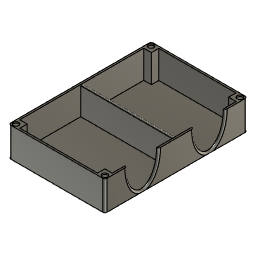
Wingspan - Birdcards (Autodesk Fusion 360 design; units mm, degrees)
Autodesk Fusion 360 part; units mm, degrees
sketch "Skizze1" plane through (0, 0, 0) normal (0, 0, 1) x (1, 0, 0)
  line L0 (0, 0) -> (91.5, 0)
  line L1 (91.5, 0) -> (91.5, 135.5)
  line L2 (91.5, 135.5) -> (0, 135.5)
  line L3 (0, 135.5) -> (0, 0)
  line L4 (1.75, 126.75) -> (89.75, 126.75)
  line L5 (89.75, 126.75) -> (89.75, 68.75)
  line L6 (89.75, 68.75) -> (1.75, 68.75)
  line L7 (1.75, 68.75) -> (1.75, 126.75)
  line L8 (0, 135.5) -> (7, 135.5)
  line L9 (7, 135.5) -> (7, 128.5)
  line L10 (7, 128.5) -> (0, 128.5)
  line L11 (0, 128.5) -> (0, 135.5)
  circle A0 centre (3.5, 132) radius 2.65
  line L12 (1.75, 66.75) -> (89.75, 66.75)
  line L13 (89.75, 66.75) -> (89.75, 8.75)
  line L14 (89.75, 8.75) -> (1.75, 8.75)
  line L15 (1.75, 8.75) -> (1.75, 66.75)
  line L16 (0, 0) -> (7, 0)
  line L17 (7, 0) -> (7, 7)
  line L18 (7, 7) -> (0, 7)
  line L19 (0, 7) -> (0, 0)
  circle A1 centre (3.5, 3.5) radius 2.65
  line L20 (91.5, 0) -> (84.5, 0)
  line L21 (84.5, 0) -> (84.5, 7)
  line L22 (84.5, 7) -> (91.5, 7)
  line L23 (91.5, 7) -> (91.5, 0)
  circle A2 centre (88, 3.5) radius 2.65
  line L24 (91.5, 135.5) -> (84.5, 135.5)
  line L25 (84.5, 135.5) -> (84.5, 128.5)
  line L26 (84.5, 128.5) -> (91.5, 128.5)
  line L27 (91.5, 128.5) -> (91.5, 135.5)
  circle A3 centre (88, 132) radius 2.65
  line L28 (9, 126.75) -> (82.5, 126.75)
  line L29 (82.5, 126.75) -> (82.5, 133.75)
  line L30 (82.5, 133.75) -> (9, 133.75)
  line L31 (9, 133.75) -> (9, 126.75)
  line L32 (8.75, 8.75) -> (82.75, 8.75)
  line L33 (82.75, 8.75) -> (82.75, 1.75)
  line L34 (82.75, 1.75) -> (8.75, 1.75)
  line L35 (8.75, 1.75) -> (8.75, 8.75)
  dimension "d3" = 88
  dimension "d4" = 58
  dimension "d5" = 7
  dimension "d6" = 7
  dimension "d7" = 5.3
  dimension "d9" = 3.5
  dimension "d10" = 3.5
  dimension "d11" = 1.75
  dimension "d12" = 1.75
  dimension "d13" = 88
  dimension "d14" = 58
  dimension "d15" = 2
  dimension "d16" = 1.75
  dimension "d17" = 8.75
  dimension "d18" = 8.75
  dimension "d19" = 135.5
  dimension "d20" = 7
  dimension "d21" = 7
  dimension "d22" = 5.3
  dimension "d24" = 3.5
  dimension "d25" = 3.5
  dimension "d26" = 1.75
  dimension "d27" = 7
  dimension "d28" = 7
  dimension "d29" = 5.3
  dimension "d30" = 3.5
  dimension "d32" = 3.5
  dimension "d33" = 7
  dimension "d34" = 7
  dimension "d35" = 5.3
  dimension "d36" = 3.5
  dimension "d37" = 3.5
  dimension "d38" = 2
  dimension "d39" = 2
  dimension "d40" = 1.75
  dimension "d41" = 1.75
  dimension "d42" = 1.75
  dimension "d43" = 1.75
  constraint horizontal L0
  constraint vertical L1
  constraint horizontal L2
  constraint vertical L3
  constraint coincident L0.start L3.end
  constraint horizontal L4
  constraint vertical L5
  constraint horizontal L6
  constraint vertical L7
  constraint horizontal L8
  constraint vertical L9
  constraint horizontal L10
  constraint vertical L11
  constraint horizontal L12
  constraint vertical L13
  constraint horizontal L14
  constraint vertical L15
  constraint horizontal L16
  constraint vertical L17
  constraint horizontal L18
  constraint vertical L19
  constraint horizontal L20
  constraint vertical L21
  constraint horizontal L22
  constraint vertical L23
  constraint horizontal L24
  constraint vertical L25
  constraint horizontal L26
  constraint vertical L27
  constraint horizontal L28
  constraint vertical L29
  constraint horizontal L30
  constraint vertical L31
  constraint coincident L4 L28.start
  constraint horizontal L32
  constraint vertical L33
  constraint horizontal L34
  constraint vertical L35
  constraint coincident L14 L32.start
  measures "d3" distance of L4.start L4.end
  measures "d4" distance of L4.start L6.end
  measures "d5" distance of L2.end L8.end
  measures "d6" distance of L2.end L10.end
  measures "d7" diameter of A0
  measures "d9" distance of L10 A0.centre
  measures "d10" distance of L11 A0.centre
  measures "d11" distance of L3 L7
  measures "d12" distance of L4 L10
  measures "d13" distance of L12.start L12.end
  measures "d14" distance of L12.start L14.end
  measures "d16" distance of L3 L15
  measures "d17" distance of L2 L4
  measures "d18" distance of L0 L14
  measures "d19" distance of L0 L2
  measures "d20" distance of L0.start L16.end
  measures "d21" distance of L0.start L18.end
  measures "d22" diameter of A1
  measures "d24" distance of L16 A1.centre
  measures "d25" distance of L3 A1.centre
  measures "d26" distance of L1 L13
  measures "d27" distance of L0.end L20.end
  measures "d28" distance of L0.end L22.end
  measures "d29" diameter of A2
  measures "d30" distance of L1 A2.centre
  measures "d32" distance of L0 A2.centre
  measures "d33" distance of L1.end L24.end
  measures "d34" distance of L1.end L26.end
  measures "d35" diameter of A3
  measures "d36" distance of L24 A3.centre
  measures "d37" distance of L27 A3.centre
  measures "d38" distance of L9 L31
  measures "d39" distance of L25 L29
  measures "d40" distance of L2 L30
  measures "d41" distance of L0 L34
  measures "d42" distance of L17 L35
  measures "d43" distance of L21 L33
sketch "Skizze2" plane through (0, 0, 0) normal (0, 0, 1) x (1, 0, 0)
  line L0 (0, 0) -> (91.5, 0)
  line L1 (91.5, 0) -> (91.5, 135.5)
  line L2 (91.5, 135.5) -> (0, 135.5)
  line L3 (0, 135.5) -> (0, 0)
  dimension "d44" = 91.5
  dimension "d45" = 135.5
  constraint horizontal L0
  constraint vertical L1
  constraint horizontal L2
  constraint vertical L3
  constraint coincident L0.start L3.end
  measures "d44" distance of L0.start L0.end
  measures "d45" distance of L0.start L2.end
extrude "Extrusion7" add sketch "Skizze2" against normal blind 28
extrude "Extrusion8" cut sketch "Skizze1" against normal blind 26.5 contours L4 L5 L6 L7 L28 | L4 L28 L29 L30 L31 | L12 L13 L14 L15 L32 | L14 L32 L33 L34 L35
extrude "Extrusion9" cut sketch "Skizze1" against normal blind 1.1 contours A0 | A1 | A2 | A3
extrude "Extrusion11" cut 3 faces at (87.1265, 132.8635, -1.1) (3.4053, 132.6906, -1.1) (88.066, 2.6191, -1.1) along direction (0, 0, -1) blind 0.1
sketch "Skizze5" plane through (91.5, 0, 0) normal (1, 0, 0) x (0, 1, 0)
  line L0 (135.5, 0) -> (0, 0)
  line L1 (0, 0) -> (0, -28)
  line L2 (0, -28) -> (135.5, -28)
  line L3 (135.5, -28) -> (135.5, 0)
  ellipse E0 centre (36, 0) end of major axis (51, 0) minor radius 26.5
  line L4 (21, 0) -> (51, 0)
  line L5 (36, -26.5) -> (36, 26.5)
  ellipse E1 centre (99.5, 0) end of major axis (114.5, 0) minor radius 26.5
  line L6 (84.5, 0) -> (114.5, 0)
  line L7 (99.5, -26.5) -> (99.5, 26.5)
  dimension "d96" = 30
  dimension "d97" = 53
  dimension "d98" = 36
  dimension "d99" = 30
  dimension "d100" = 53
  dimension "d101" = 36
  constraint coincident L0 E0.centre
  constraint parallel L0 L4
  constraint coincident E0 L4.start
  constraint coincident E0 L4.end
  constraint coincident E0 L5.start
  constraint coincident E0 L5.end
  constraint coincident L0 E1.centre
  constraint parallel L0 L6
  constraint coincident E1 L6.start
  constraint coincident E1 L6.end
  constraint coincident E1 L7.start
  constraint coincident E1 L7.end
  measures "d96" distance of E0
  measures "d98" distance of L1 E0.centre
  measures "d99" distance of E1
  measures "d101" distance of L3 E1.centre
extrude "Extrusion12" cut sketch "Skizze5" against normal blind 26 contours L0 E1 L6 L7 | L0 E1 L6 L7 | L0 E0 L4 L5 | L0 E0 L4 L5 picked at (102.3495, -16.0918) picked at (96.5218, -15.9287) picked at (38.8495, -16.0918) picked at (33.0218, -15.9287)
fillet "Abrundung8" radius 2 4 edges at (91.5, 0, -14) (91.5, 135.5, -14) (0, 135.5, -14) (0, 0, -14)
fillet "Abrundung9" radius 2 2 edges at (91.5, 36, -26.5) (91.5, 99.5, -26.5)
fillet "Abrundung10" radius 1 2 edges at (45.75, 66.75, 0) (45.75, 68.75, 0)
sketch "Skizze4" plane through (91.5, 0, 0) normal (1, 0, 0) x (0, 1, 0)
  line L0 (135.5, 0) -> (0, 0)
  line L1 (0, 0) -> (0, -28)
  line L2 (0, -28) -> (135.5, -28)
  line L3 (135.5, -28) -> (135.5, 0)
  ellipse E0 centre (98, 0) end of major axis (111, 0) minor radius 26.5
  line L4 (85, 0) -> (111, 0)
  line L5 (98, -26.5) -> (98, 26.5)
  ellipse E1 centre (37.5, 0) end of major axis (50.5, 0) minor radius 26.5
  line L6 (24.5, 0) -> (50.5, 0)
  line L7 (37.5, -26.5) -> (37.5, 26.5)
  dimension "d80" = 26
  dimension "d81" = 53
  dimension "d82" = 37.5
  dimension "d83" = 26
  dimension "d84" = 53
  dimension "d85" = 37.5
  constraint coincident L0 E0.centre
  constraint parallel L0 L4
  constraint coincident E0 L4.start
  constraint coincident E0 L4.end
  constraint coincident E0 L5.start
  constraint coincident E0 L5.end
  constraint coincident L0 E1.centre
  constraint parallel L0 L6
  constraint coincident E1 L6.start
  constraint coincident E1 L6.end
  constraint coincident E1 L7.start
  constraint coincident E1 L7.end
  measures "d80" distance of E0
  measures "d82" distance of L3 L5
  measures "d83" distance of E1
  measures "d85" distance of L1 L7
extrude "Extrusion10" [suppressed]
fillet "Abrundung5" [suppressed]
fillet "Abrundung6" [suppressed]
fillet "Abrundung7" [suppressed]
extrude "Extrusion1" [suppressed]
extrude "Extrusion2" [suppressed]
extrude "Extrusion3" [suppressed]
extrude "Extrusion4" [suppressed]
extrude "Extrusion5" [suppressed]
sketch "Skizze3" plane through (91.5, 0, 0) normal (1, 0, 0) x (0, 1, 0)
  line L0 (135.5, 0) -> (0, 0)
  line L1 (0, 0) -> (0, -27.75)
  line L2 (0, -27.75) -> (135.5, -27.75)
  line L3 (135.5, -27.75) -> (135.5, 0)
  line L4 (28.5, 0) -> (44.5, 0)
  line L5 (44.5, 0) -> (44.5, -26)
  line L6 (44.5, -26) -> (28.5, -26)
  line L7 (28.5, -26) -> (28.5, 0)
  line L8 (91, 0) -> (107, 0)
  line L9 (107, 0) -> (107, -26)
  line L10 (107, -26) -> (91, -26)
  line L11 (91, -26) -> (91, 0)
  dimension "d56" = 16
  dimension "d57" = 26
  dimension "d58" = 28.5
  dimension "d59" = 16
  dimension "d60" = 26
  dimension "d61" = 28.5
  constraint horizontal L4
  constraint vertical L5
  constraint horizontal L6
  constraint vertical L7
  constraint coincident L0 L4.start
  constraint horizontal L8
  constraint vertical L9
  constraint horizontal L10
  constraint vertical L11
  constraint coincident L0 L8.start
  measures "d56" distance of L4.start L4.end
  measures "d57" distance of L4.start L6.end
  measures "d58" distance of L1 L7
  measures "d59" distance of L8.start L8.end
  measures "d60" distance of L8.start L10.end
  measures "d61" distance of L3 L9
extrude "Extrusion6" [suppressed]
fillet "Abrundung1" [suppressed]
fillet "Abrundung2" [suppressed]
fillet "Abrundung3" [suppressed]
fillet "Abrundung4" [suppressed]
equation "d46 = -26 mm - 1.75 mm"
equation "d58 = ( 57 / 2 ) * 1 mm"
equation "d61 = ( 57 / 2 ) * 1 mm"
equation "d74 = -28 mm + 1.5 mm"
equation "d81 = 56 mm - 1.5 mm * 2"
equation "d84 = 28 * 2 mm - 3 mm"
equation "d97 = ( ( 28 * 2 ) * 1 mm ) - 3 mm"
